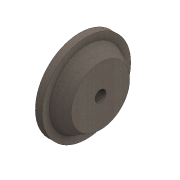
# Autodesk Inventor part: wheel
Saved by Autodesk Inventor 2020 (Build 240168000, 168)
## iProperties
Created: 2021-06-22
Part Number: wheel
Material: Generic
Document SubType Name: Modeling
Designer: Aidan Lee
Density: 1 g/cm^3
Appearance: Walnut
Author: Aidan Lee
Autodesk Inventor part; units mm, degrees
ref_plane "YZ Plane" through (0, 0, 0) normal (1, 0, 0) x (0, 1, 0)
ref_plane "XZ Plane" through (0, 0, 0) normal (0, 1, 0) x (-1, 0, 0)
ref_plane "XY Plane" through (0, 0, 0) normal (0, 0, 1) x (1, 0, 0)
sketch "Sketch1" plane through (0, 0, 0) normal (0, 0, 1) x (1, 0, 0)
  line L0 (-67.5, 66.7321) -> (-62.5, 66.7321) construction
  line L1 (-62.5, 66.7321) -> (-62.5, 3.2679) construction
  line L2 (-62.5, 3.2679) -> (-67.5, 3.2679) construction
  line L3 (-67.5, 3.2679) -> (-67.5, 66.7321) construction
  line L4 (-62.5, 61.7321) -> (-52.5, 55.9585) construction
  line L5 (-52.5, 55.9585) -> (-52.5, 14.0415) construction
  line L6 (-52.5, 14.0415) -> (-62.5, 8.2679) construction
  line L7 (-56.5, 10) -> (-56.5, 0) construction
  line L8 (-59.5, 10) -> (-59.5, 60) construction
  line L9 (-62.5, 61.7321) -> (-52.5, 55.9585)
  line L10 (-62.5, 61.7321) -> (-62.5, 66.7321)
  line L11 (-67.5, 66.7321) -> (-62.5, 66.7321)
  line L12 (-52.5, 31) -> (-166.5, 31) construction
  line L13 (-166.5, 31) -> (-166.5, 39) construction
  line L14 (-166.5, 39) -> (-52.5, 39) construction
  line L15 (-52.5, 39) -> (-52.5, 31) construction
  line L16 (0, 0) -> (-219, 0) construction
  line L17 (-219, 0) -> (-219, -18) construction
  line L18 (-219, -18) -> (0, -18) construction
  line L19 (0, -18) -> (0, 0) construction
  line L20 (-109.5, -55.8166) -> (-109.5, -71.0824) construction
  line L21 (-67.5, 66.7321) -> (-67.5, 39)
  line L22 (-52.5, 39) -> (-67.5, 39)
  line L23 (-52.5, 39) -> (-52.5, 55.9585)
  line L24 (-52.5, 35) -> (-67.5, 35) construction
  line L25 (-166.5, 55.9585) -> (-166.5, 14.0415) construction
  line L26 (-159.5, 10) -> (-159.5, 60) construction
  line L27 (-156.5, 66.7321) -> (-156.5, 3.2679) construction
  line L28 (-151.5, 3.2679) -> (-151.5, 66.7321) construction
  line L29 (-151.5, 66.7321) -> (-156.5, 66.7321) construction
  line L30 (-156.5, 61.7321) -> (-166.5, 55.9585) construction
  line L31 (-166.5, 14.0415) -> (-156.5, 8.2679) construction
  line L32 (-159.5, 10) -> (-162.5, 10) construction
  line L33 (-156.5, 3.2679) -> (-151.5, 3.2679) construction
  line L34 (-156.5, 61.7321) -> (-166.5, 55.9585) construction
  line L35 (-156.5, 61.7321) -> (-156.5, 66.7321) construction
  line L36 (-151.5, 66.7321) -> (-156.5, 66.7321) construction
  line L37 (-166.5, 39) -> (-166.5, 31) construction
  line L38 (-166.5, 39) -> (-151.5, 39) construction
  line L39 (-166.5, 39) -> (-166.5, 55.9585) construction
  line L40 (-166.5, 35) -> (-151.5, 35) construction
  line L41 (-56.5, 10) -> (-59.5, 10) construction
  line L42 (-59.5, 10) -> (-59.5, 0) construction
  line L43 (-59.5, 0) -> (-56.5, 0) construction
  point P0 (-62.5, 35)
  point P1 (-109.5, -63.4495)
  point P2 (-109.5, -18)
  point P3 (-109.5, 31)
  point P4 (-156.5, 35)
  dimension "d0" = 60
  dimension "d1" = 5
  dimension "d4" = 5
  dimension "d5" = 10
  dimension "d6" = 50
  dimension "d7" = 4
  dimension "d9" = 18
  dimension "d10" = 219
  dimension "d12" = 114
  dimension "d14" = 8
  dimension "d15" = 3
  dimension "d16" = 3
  dimension "d17" = 100
  dimension "d18" = 84
  constraints: 89 end point, 14 symmetric about line, 13 point on line, 7 midpoint, 7 parallel, 7 perpendicular, 5 horizontal, 3 horizontal alignment, 2 collinear, 2 vertical, 2 vertical alignment, 1 equal length
  measures "d0" angle of L1 L6
  measures "d1" distance of L3.end L1.start
  measures "d4" distance from line of L6.end L2
  measures "d5" distance of L7.start L7.end
  measures "d6" distance of L8.start L8.end
  measures "d7" distance between parallel lines of L5 L7
  measures "d9" distance of L16.start L18.end
  measures "d10" distance of L17.end L18.end
  measures "d12" distance of L13.end L14.end
  measures "d14" distance of L12.end L13.end
  measures "d15" distance of L42.end L7.end
  measures "d16" distance between parallel lines of L42 L1
  measures "d17" distance from line of L26.start L42
  measures "d18" distance between parallel lines of L3 L28
revolve "Revolution1" add sketch "Sketch1" angle 360 about axis through (-52.5, 35, 0) along (-1, 0, 0)
body "Solid1"
